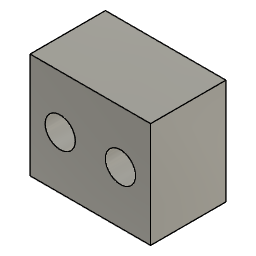
LED Frame v12 (Autodesk Fusion 360 archive; units mm, degrees)
design "LED Holder"
Autodesk Fusion 360 part; units mm, degrees
sketch "Base" plane through (0, 0, 0) normal (0, 0, 1) x (1, 0, 0)
  line L0 (0, 0) -> (8, 0)
  line L1 (8, 0) -> (8, 5)
  line L2 (8, 5) -> (0, 5)
  line L3 (0, 5) -> (0, 0)
  dimension "d45" = 8
  dimension "d46" = 5
  constraint horizontal L0
  constraint vertical L1
  constraint horizontal L2
  constraint vertical L3
  constraint coincident L0.start L3.end
  measures "d45" distance of L0.start L0.end
  measures "d46" distance of L0.start L2.end
extrude "Extrude7" add sketch "Base" along normal blind 7
sketch "Holes" plane through (0, 0, 0) normal (0, -1, 0) x (1, 0, 0)
  line L0 (0, 0) -> (8, 0)
  line L1 (8, 0) -> (8, 7)
  line L2 (8, 7) -> (0, 7)
  line L3 (0, 7) -> (0, 0)
  circle A0 centre (2, 3.5) radius 1
  line L4 (4, 7) -> (4, 0) construction
  circle A1 centre (6, 3.5) radius 1
  line L5 (0, 3.5) -> (8, 3.5) construction
  dimension "d50" = 2
  dimension "d51" = 8
  dimension "d55" = 2
  constraint midpoint L2 L4.start
  constraint midpoint L0 L4.end
  constraint symmetric A0 L4 A1
  constraint midpoint L3 L5.start
  constraint midpoint L1 L5.end
  constraint coincident A0.centre L5
  measures "d50" diameter of A0
  measures "d51" distance of L1.end L2.end
  measures "d55" distance of A0.centre L4
extrude "Extrude8" cut sketch "Holes" against normal through all contours A0 | A1
equation "hole_d = 2 mm"
equation "d50 = hole_d"
equation "d40 = ( base_width - lead_holder_delta_width ) / 3"
equation "d41 = d40"
equation "d43 = base_depth + lead_hole_pos_z"
equation "d44 = d43"
